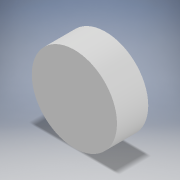
# Autodesk Inventor part: schablone
Saved by Autodesk Inventor 2020.2 (Build 242310000, 310)
## iProperties
Created: 2021-11-04
Part Number: schablone
Material: Generisch
Document SubType Name: Modeling
Designer: johan
Density: 1 g/cm^3
Appearance: Vorgabe
Author: johan
Autodesk Inventor part; units mm, degrees
ref_plane "YZ Plane" through (0, 0, 0) normal (1, 0, 0) x (0, 1, 0)
ref_plane "XZ Plane" through (0, 0, 0) normal (0, 1, 0) x (-1, 0, 0)
ref_plane "XY Plane" through (0, 0, 0) normal (0, 0, 1) x (1, 0, 0)
sketch "Skizze1" plane through (0, 0, 0) normal (0, 0, 1) x (1, 0, 0)
  circle A0 centre (0, 0) radius 13.7
  circle A1 centre (0, 0) radius 15
  dimension "d0" = 27.4
  dimension "d1" = 30
  constraints: 2 centre point, 2 coincident
  measures "d0" diameter of A0
  measures "d1" diameter of A1
extrude "Extrusion1" add sketch "Skizze1" along normal blind 2
sketch "Skizze2" plane through (0, 0, 2) normal (0, 0, 1) x (1, 0, 0)
  circle A0 centre (0, 0) radius 15
  dimension "d4" = 30
  constraints: 1 centre point, 1 coincident
  measures "d4" diameter of A0
extrude "Extrusion2" add sketch "Skizze2" along normal blind 9
sketch "Skizze3" plane through (0, 0, 2) normal (0, 0, -1) x (-1, 0, 0)
  circle A0 centre (3.25, 0) radius 2.1
  circle A1 centre (-3.25, 0) radius 3
  point P0 (0, 0)
  dimension "d7" = 4.2
  dimension "d8" = 6
  dimension "d10" = 3.25
  dimension "d11" = 3.25
  dimension "d12" = 6.5
  constraints: 2 centre point
  measures "d7" diameter of A0
  measures "d8" diameter of A1
  measures "d10" distance of point (0, 0) A0.centre
  measures "d11" distance of A1.centre point (0, 0)
  measures "d12" distance of A1.centre A0.centre
extrude "Extrusion3" cut sketch "Skizze3" against normal blind 1.2
sketch "Skizze4" plane through (3.25, 0, 3.2) normal (0, 0, -1) x (-1, 0, 0)
  circle A0 centre (0, 0) radius 2.5
  circle A1 centre (6.5, 0) radius 2.1 projected
  circle A2 centre (6.5, 0) radius 1.9
  point P0 (3.25, 0)
  dimension "d15" = 5
  dimension "d16" = 3.8
  dimension "d17" = 6.5
  dimension "d18" = 3.25
  constraints: 2 centre point, 1 coincident
  measures "d15" diameter of A0
  measures "d16" diameter of A2
  measures "d17" distance of A1.centre A0.centre
  measures "d18" distance of point (3.25, 0) A0.centre
extrude "Extrusion4" cut sketch "Skizze4" against normal blind 3.4 contours A0 | A2
sketch "Skizze5" plane through (3.25, 0, 6.6) normal (0, 0, -1) x (-1, 0, 0)
  circle A0 centre (6.5, 0) radius 1.9 projected
  circle A1 centre (6.5, 0) radius 1.6
  circle A2 centre (0, 0) radius 2.5
  point P0 (3.25, 0)
  dimension "d21" = 3.2
  dimension "d22" = 5
  dimension "d23" = 6.5
  dimension "d24" = 3.25
  constraints: 2 centre point, 1 coincident
  measures "d21" diameter of A1
  measures "d22" diameter of A2
  measures "d23" distance of A0.centre A2.centre
  measures "d24" distance of point (3.25, 0) A2.centre
extrude "Extrusion5" cut sketch "Skizze5" against normal blind 4 contours A1 | A2
